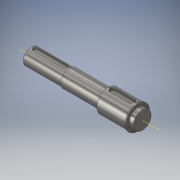
# Autodesk Inventor part: GonjenoVratilo
Saved by Autodesk Inventor 2018 (Build 220112000, 112)
## iProperties
Created: 2018-11-17
Part Number: GonjenoVratilo
Material: Steel, Carbon
Document SubType Name: Modeling
Designer: Kristijan
Density: 7.85 g/cm^3
Appearance: Semi-Polished
Mass: 11718.7 g
Surface Area: 1017.01 cm^2
Volume: 1492.82 cm^3
Author: Kristijan
Autodesk Inventor part; units mm, degrees
ref_plane "YZ Plane" through (0, 0, 0) normal (1, 0, 0) x (0, 1, 0)
sketch "Sketch1" plane through (0, 0, 0) normal (0, 0, 1) x (1, 0, 0)
  point P0 (0, 0)
sketch "Sketch2" plane through (0, 0, 0) normal (0, 0, 1) x (1, 0, 0)
  line L0 (0, 0) -> (0, 29)
  line L1 (1, 30) -> (140, 30)
  line L2 (140, 30) -> (140, 32.5)
  line L3 (140, 32.5) -> (175, 32.5)
  line L4 (280, 37.5) -> (280, 42)
  line L5 (280, 42) -> (384, 42)
  line L6 (384, 42) -> (384, 44)
  line L7 (384, 44) -> (389, 44)
  line L8 (389, 44) -> (389, 39.5)
  line L9 (300, 32.5) -> (405, 32.5)
  line L10 (406, 31.5) -> (406, 0)
  line L11 (406, 0) -> (0, 0)
  line L12 (0, 29) -> (1, 30)
  line L13 (405, 32.5) -> (406, 31.5)
  line L14 (-81.2, 0) -> (487.2, 0) projected
  line L15 (389, 39.5) -> (389, 32.5)
  line L16 (389, 32.5) -> (300, 32.5)
  line L17 (280, 37.5) -> (280, 32.5)
  line L18 (280, 32.5) -> (175, 32.5)
  point P0 (0, 30)
  point P1 (406, 32.5)
  dimension "d0" = 30
  dimension "d1" = 140
  dimension "d2" = 32.5
  dimension "d3" = 140
  dimension "d4" = 104
  dimension "d5" = 5
  dimension "d6" = 17
  dimension "d7" = 32.5
  dimension "d8" = 42
  dimension "d9" = 2
  dimension "d10" = 1
  dimension "d11" = 45
  dimension "d12" = 1
  dimension "d13" = 45
  constraints: 36 end point, 11 perpendicular, 8 point on line, 4 vertical, 1 horizontal
  measures "d0" distance between parallel lines of L11 L1
  measures "d1" distance of point (0, 30) L1.end
  measures "d2" distance between parallel lines of L11 L3
  measures "d3" distance of L2.end L17.end
  measures "d4" distance of L4.end L5.end
  measures "d5" distance of L6.end L7.end
  measures "d6" distance of L15.end point (406, 32.5)
  measures "d7" distance between parallel lines of L11 L9
  measures "d8" distance between parallel lines of L11 L5
  measures "d9" distance of L5.end L6.end
  measures "d10" distance of L0.end point (0, 30)
  measures "d11" angle of L0 L12
  measures "d12" distance of L9.end point (406, 32.5)
  measures "d13" angle of L9 L13
revolve "Revolution1" add sketch "Sketch2" angle 360 about axis through (-10, 0, 0) along (1, 0, 0)
ref_plane "Work Plane1" through (70.5, 30, 0) normal (0, 1, 0) x (-1, 0, 0)
ref_plane "Work Plane2" through (332, 42, 0) normal (0, 1, 0) x (-1, 0, 0)
sketch "Sketch3" plane through (70.5, 30, 0) normal (0, 1, 0) x (-1, 0, 0)
  line L0 (54, 0) -> (-53, 0) construction
  line L1 (54, 9) -> (-53, 9)
  line L2 (-53, -9) -> (54, -9)
  arc A0 (54, -9) -> (54, 9) centre (54, 0) ccw
  arc A1 (-53, 9) -> (-53, -9) centre (-53, 0) ccw
  line L3 (-69.5, 32.5) -> (-69.5, -32.5) projected
  line L4 (0.5, -9) -> (0.5, 9) construction
  line L5 (70.5, 0) -> (-69.5, 0) construction
  line L6 (0.5, 0) -> (0.5, 9) construction
  line L7 (70.5, 29) -> (70.5, -29) construction
  point P0 (0.5, 0)
  dimension "d16" = 125
  dimension "d18" = 9
  dimension "d30" = 7.5
  dimension "d31" = 7.5
  constraints: 14 end point, 7 midpoint, 4 point on circle, 4 tangent, 2 centre point, 1 horizontal, 1 parallel, 1 perpendicular
  measures "d18" radius of A0
  measures "d30" distance edge to line of A1 L3
  measures "d31" distance edge to line of A0 L7
extrude "Extrusion1" cut sketch "Sketch3" against normal blind 7
sketch "Sketch4" plane through (332, 42, 0) normal (0, 1, 0) x (-1, 0, 0)
  line L0 (34, 0) -> (-34, 0) construction
  line L1 (34, -11) -> (-34, -11)
  line L2 (-34, 11) -> (34, 11)
  arc A0 (34, -11) -> (34, 11) centre (34, 0) ccw
  arc A1 (-34, 11) -> (-34, -11) centre (-34, 0) ccw
  line L3 (-52, 44) -> (-52, -44) projected
  line L4 (52, 42) -> (52, -42) projected
  line L5 (52, 42) -> (52, -42) construction
  line L6 (-52, 42) -> (-52, -42) construction
  line L7 (413.8, 0) -> (-155.3, 0) construction
  line L8 (-52, 0) -> (52, 0) construction
  line L9 (0, 11) -> (0, -11) construction
  line L10 (52, 42) -> (-52, 42) construction
  line L11 (0, 42) -> (0, -42) construction
  point P0 (332, 0)
  point P1 (0, 0)
  point P2 (0, 0)
  dimension "d22" = 11
  dimension "d32" = 90
  constraints: 14 end point, 8 midpoint, 4 point on circle, 4 tangent, 2 centre point, 2 point on line, 1 horizontal, 1 parallel, 1 perpendicular
  measures "d22" radius of A0
extrude "Extrusion2" cut sketch "Sketch4" against normal blind 9
chamfer "Chamfer1" distance 1 angle 45 1 edges at (389, -44, 0) measured on face at (389, 1.3058, -39.927)
chamfer "Chamfer2" distance 1 angle 60 1 edges at (280, -42, 0) measured on face at (349.3333, 24.8095, 33.8893)
fillet "Fillet1" radius 1 1 edges at (280, -32.5, 0)
fillet "Fillet2" radius 1 1 edges at (140, -30, 0)
fillet "Fillet3" radius 1 1 edges at (389, -32.5, 0)
equation "\"d7\" = d2"
equation "\"d12\" = d10"
equation "\"d13\" = d11"
body "Solid1"
